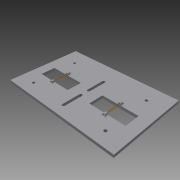
# Autodesk Inventor part: Down
Saved by Autodesk Inventor 2015 (Build 190159000, 159)
## iProperties
Created: 2018-12-21
Part Number: Down
Material: Типовые
Document SubType Name: Modeling
Designer: kostya
Density: 1 g/cm^3
Appearance: По умолчанию
Author: kostya
Autodesk Inventor part; units mm, degrees
ref_plane "YZ Plane" through (0, 0, 0) normal (1, 0, 0) x (0, 1, 0)
ref_plane "XZ Plane" through (0, 0, 0) normal (0, 1, 0) x (-1, 0, 0)
sketch "Эскиз1" plane through (0, 0, 0) normal (0, 0, 1) x (1, 0, 0)
  line L0 (-100, -75) -> (100, -75)
  line L1 (100, -75) -> (100, 75)
  line L2 (100, 75) -> (-100, 75)
  line L3 (-100, 75) -> (-100, -75)
  line L4 (-100, -75) -> (100, 75) construction
  line L5 (100, -75) -> (-100, 75) construction
  point P0 (0, 0)
  dimension "d0" = 200
  dimension "d1" = 150
  constraints: 12 end point, 2 midpoint, 2 parallel, 1 horizontal, 1 perpendicular
  measures "d0" distance of L2.end L1.end
  measures "d1" distance of L1.end L0.end
extrude "Выдавливание1" add sketch "Эскиз1" along normal blind 5
sketch "Эскиз2" plane through (0, 0, 5) normal (0, 0, 1) x (1, 0, 0)
  line L0 (-100, -75) -> (100, -75) projected
  line L1 (100, -75) -> (100, 75) projected
  line L2 (100, 75) -> (-100, 75) projected
  line L3 (-100, 75) -> (-100, -75) projected
  line L4 (100, 75) -> (-100, 75) construction
  line L5 (0, 75) -> (0, -75) construction
  line L6 (-100, 0) -> (100, 0) construction
  line L7 (100, -75) -> (100, 75) construction
  line L8 (-100, -12.5) -> (100, -12.5) construction
  line L9 (100, -12.5) -> (100, 12.5) construction
  line L10 (100, 12.5) -> (-100, 12.5) construction
  line L11 (-100, 12.5) -> (-100, -12.5) construction
  line L12 (-100, -12.5) -> (100, 12.5) construction
  line L13 (100, -12.5) -> (-100, 12.5) construction
  line L14 (-100, 0) -> (0, 0) construction
  line L15 (-51.2124, 75) -> (-51.2124, -75) construction
  line L16 (-100, -75) -> (100, -75) construction
  line L17 (0, 0) -> (100, 0) construction
  line L18 (50, 75) -> (50, -75) construction
  line L19 (-81.2124, -12.5) -> (-21.2124, -12.5)
  line L20 (-21.2124, -12.5) -> (-21.2124, 12.5)
  line L21 (-21.2124, 12.5) -> (-81.2124, 12.5)
  line L22 (-81.2124, 12.5) -> (-81.2124, -12.5)
  line L23 (-81.2124, -12.5) -> (-21.2124, 12.5) construction
  line L24 (-21.2124, -12.5) -> (-81.2124, 12.5) construction
  line L25 (81.2124, -12.5) -> (21.2124, -12.5)
  line L26 (21.2124, -12.5) -> (21.2124, 12.5)
  line L27 (21.2124, 12.5) -> (81.2124, 12.5)
  line L28 (81.2124, 12.5) -> (81.2124, -12.5)
  point P0 (-51.2124, 0)
  dimension "d4" = 25
  dimension "d5" = 60
  constraints: 44 end point, 9 midpoint, 6 point on line, 4 parallel, 4 perpendicular, 4 symmetric about line, 2 collinear, 2 horizontal
  measures "d4" distance of L9.end L8.end
  measures "d5" distance of L21.end L20.end
extrude "Выдавливание2" cut sketch "Эскиз2" against normal blind 5 contours L22 L21 L20 L19 | L25 L26 L27 L28
sketch "Эскиз3" plane through (-81.2124, 12.5, 5) normal (0, -1, 0) x (1, 0, 0)
  line L0 (0, 0) -> (60, 0) projected
  line L1 (30, 0) -> (30, 14.9537) construction
  line L2 (30, 0) -> (40, 0) construction
  line L3 (30, 0) -> (35, 0) construction
  line L4 (30, 0) -> (25, 0) construction
  line L5 (25, 0) -> (35, 0) construction
  line L6 (25, 0) -> (35, 0)
  line L7 (30, 0) -> (30, 3) construction
  circle A0 centre (30, 1.5) radius 1.5
  arc A1 (32.3946, 0.7816) -> (27.6054, 0.7816) centre (30, 1.5) ccw
  line L8 (35, 0) -> (32.3946, 0.7816)
  line L9 (25, 0) -> (27.6054, 0.7816)
  point P0 (81.2124, -5)
  dimension "d8" = 10
  dimension "d9" = 5
  dimension "d10" = 5
  dimension "d11" = 3
  dimension "d12" = 1
  constraints: 18 end point, 3 midpoint, 3 point on line, 2 collinear, 2 point on circle, 1 centre point, 1 vertical, 1 vertical alignment, 2 other
  measures "d8" distance of L1.start L2.end
  measures "d9" distance of L1.start L3.end
  measures "d10" distance of L1.start L4.end
  measures "d11" distance of L1.start L7.end
extrude "Выдавливание3" add sketch "Эскиз3" against normal blind 5
mirror "Зеркальное отражение1" about plane through (0, 0, 0) normal (0, 1, 0) of "Выдавливание3"
sketch "Эскиз4" plane through (-81.2124, 12.5, 0) normal (0, -1, 0) x (1, 0, 0)
  circle A0 centre (30, 6.5) radius 1.5 projected
  point P0 (81.2124, 0)
surface extrude "ВыдавПврх1" sketch "Эскиз4" along normal up to next shown yes curves A0
boundary_patch "Участок поверхности1"
boundary_patch "Участок поверхности2"
ref_plane "РабПлоскость1" through (-81.2124, 0, 0) normal (0, -1, 0) x (1, 0, 0)
sketch "Эскиз6" plane through (0, 0, 5) normal (0, 0, 1) x (1, 0, 0)
  line L0 (81.2124, -12.5) -> (21.2124, -12.5) projected
  line L1 (21.2124, -12.5) -> (21.2124, 12.5) projected
  line L2 (21.2124, 12.5) -> (81.2124, 12.5) projected
  line L3 (81.2124, 12.5) -> (81.2124, -12.5) projected
  line L4 (-100, -75) -> (100, -75) projected
  line L5 (100, -75) -> (100, 75) projected
  line L6 (100, 75) -> (-100, 75) projected
  line L7 (-100, 75) -> (-100, -75) projected
  line L8 (-46.2124, -12.5) -> (-46.2124, -17.5) projected
  line L9 (-46.2124, -17.5) -> (-51.2124, -17.5) projected
  line L10 (-51.2124, -17.5) -> (-56.2124, -17.5) projected
  line L11 (-56.2124, -17.5) -> (-56.2124, -12.5) projected
  line L12 (-56.2124, -12.5) -> (-81.2124, -12.5) projected
  line L13 (-81.2124, -12.5) -> (-81.2124, 12.5) projected
  line L14 (-81.2124, 12.5) -> (-56.2124, 12.5) projected
  line L15 (-56.2124, 12.5) -> (-56.2124, 17.5) projected
  line L16 (-56.2124, 17.5) -> (-51.2124, 17.5) projected
  line L17 (-51.2124, 17.5) -> (-46.2124, 17.5) projected
  line L18 (-46.2124, 17.5) -> (-46.2124, 12.5) projected
  line L19 (-46.2124, 12.5) -> (-21.2124, 12.5) projected
  line L20 (-21.2124, 12.5) -> (-21.2124, -12.5) projected
  line L21 (-21.2124, -12.5) -> (-46.2124, -12.5) projected
  line L22 (-100, -75) -> (100, -75) construction
  line L23 (-21.2124, -75) -> (-21.2124, 75) construction
  line L24 (100, 75) -> (-100, 75) construction
  line L25 (-21.2124, 12.5) -> (-21.2124, 75) construction
  line L26 (-21.2124, 75) -> (21.2124, 75) construction
  line L27 (21.2124, 75) -> (21.2124, 12.5) construction
  line L28 (21.2124, 12.5) -> (-21.2124, 12.5) construction
  line L29 (-21.2124, 12.5) -> (-21.2124, 75) construction
  line L30 (-21.2124, -75) -> (21.2124, -75) construction
  line L31 (21.2124, -75) -> (21.2124, -12.5) construction
  line L32 (21.2124, -12.5) -> (-21.2124, -12.5) construction
  line L33 (-21.2124, -12.5) -> (-21.2124, -75) construction
  line L34 (100, -75) -> (100, 75) construction
  line L35 (-100, -7.5) -> (100, -7.5) construction
  line L36 (100, -7.5) -> (100, 7.5) construction
  line L37 (100, 7.5) -> (-100, 7.5) construction
  line L38 (-100, 7.5) -> (-100, -7.5) construction
  line L39 (-100, -7.5) -> (100, 7.5) construction
  line L40 (100, -7.5) -> (-100, 7.5) construction
  line L41 (0, 7.5) -> (0, 17.5) construction
  line L42 (0, -7.5) -> (0, -28.0993) construction
  line L43 (-2.5, -7.5) -> (-2.5, -28.0993)
  line L44 (2.5, -28.0993) -> (2.5, -7.5)
  arc A0 (2.5, -7.5) -> (-2.5, -7.5) centre (0, -7.5) ccw
  line L45 (-2.5, -28.0993) -> (-2.5, -38.0993)
  line L46 (2.5, -28.0993) -> (2.5, -38.0993)
  arc A1 (-2.5, -38.0993) -> (2.5, -38.0993) centre (0, -38.0993) ccw
  line L47 (-21.2124, 0) -> (21.2124, 0) construction
  line L48 (-2.5, 7.5) -> (-2.5, 28.0993)
  line L49 (2.5, 28.0993) -> (2.5, 7.5)
  arc A2 (-2.5, 7.5) -> (2.5, 7.5) centre (0, 7.5) ccw
  line L50 (-2.5, 28.0993) -> (-2.5, 38.0993)
  line L51 (2.5, 28.0993) -> (2.5, 38.0993)
  arc A3 (2.5, 38.0993) -> (-2.5, 38.0993) centre (0, 38.0993) ccw
  point P0 (0, 0)
  point P1 (0, -17.7997)
  point P2 (0, 17.7997)
  dimension "d24" = 15
  dimension "d25" = 10
  dimension "d27" = 10
  constraints: 56 end point, 9 symmetric about line, 8 point on circle, 7 midpoint, 7 parallel, 4 centre point, 4 perpendicular, 4 vertical, 3 horizontal, 3 point on line, 1 coincident, 1 collinear, 2 other
  measures "d24" distance of L36.end L35.end
  measures "d25" distance of L41.start L41.end
  measures "d27" distance of L43.end L45.end
extrude "Выдавливание5" cut sketch "Эскиз6" against normal blind 20 contours A0 L44 L46 A1 L45 L43 | L48 L50 A3 L51 L49 A2
mirror "Зеркальное отражение2" about plane through (0, 0, 0) normal (1, 0, 0) of "Выдавливание3", "ВыдавПврх1", "Зеркальное отражение1"
sketch "Эскиз7" plane through (0, 0, 5) normal (0, 0, 1) x (1, 0, 0)
  arc A0 (-2.5, -38.0993) -> (2.5, -38.0993) centre (0, -38.0993) ccw projected
  line L0 (-2.5, -38.0993) -> (-2.5, -7.5) projected
  arc A1 (2.5, -7.5) -> (-2.5, -7.5) centre (0, -7.5) ccw projected
  line L1 (2.5, -7.5) -> (2.5, -38.0993) projected
  arc A2 (2.5, 38.0993) -> (-2.5, 38.0993) centre (0, 38.0993) ccw projected
  line L2 (2.5, 38.0993) -> (2.5, 7.5) projected
  arc A3 (-2.5, 7.5) -> (2.5, 7.5) centre (0, 7.5) ccw projected
  line L3 (-2.5, 7.5) -> (-2.5, 38.0993) projected
  line L4 (-100, -75) -> (100, -75) projected
  line L5 (100, -75) -> (100, 75) projected
  line L6 (100, 75) -> (-100, 75) projected
  line L7 (-100, 75) -> (-100, -75) projected
  line L8 (-46.2124, -12.5) -> (-46.2124, -17.5) projected
  line L9 (-46.2124, -17.5) -> (-51.2124, -17.5) projected
  line L10 (-51.2124, -17.5) -> (-56.2124, -17.5) projected
  line L11 (-56.2124, -17.5) -> (-56.2124, -12.5) projected
  line L12 (-56.2124, -12.5) -> (-81.2124, -12.5) projected
  line L13 (-81.2124, -12.5) -> (-81.2124, 12.5) projected
  line L14 (-81.2124, 12.5) -> (-56.2124, 12.5) projected
  line L15 (-56.2124, 12.5) -> (-56.2124, 17.5) projected
  line L16 (-56.2124, 17.5) -> (-51.2124, 17.5) projected
  line L17 (-51.2124, 17.5) -> (-46.2124, 17.5) projected
  line L18 (-46.2124, 17.5) -> (-46.2124, 12.5) projected
  line L19 (-46.2124, 12.5) -> (-21.2124, 12.5) projected
  line L20 (-21.2124, 12.5) -> (-21.2124, -12.5) projected
  line L21 (-21.2124, -12.5) -> (-46.2124, -12.5) projected
  line L22 (56.2124, -12.5) -> (56.2124, -17.5) projected
  line L23 (56.2124, -17.5) -> (51.2124, -17.5) projected
  line L24 (51.2124, -17.5) -> (46.2124, -17.5) projected
  line L25 (46.2124, -17.5) -> (46.2124, -12.5) projected
  line L26 (46.2124, -12.5) -> (21.2124, -12.5) projected
  line L27 (21.2124, -12.5) -> (21.2124, 12.5) projected
  line L28 (21.2124, 12.5) -> (46.2124, 12.5) projected
  line L29 (46.2124, 12.5) -> (46.2124, 17.5) projected
  line L30 (46.2124, 17.5) -> (51.2124, 17.5) projected
  line L31 (51.2124, 17.5) -> (56.2124, 17.5) projected
  line L32 (56.2124, 17.5) -> (56.2124, 12.5) projected
  line L33 (56.2124, 12.5) -> (81.2124, 12.5) projected
  line L34 (81.2124, 12.5) -> (81.2124, -12.5) projected
  line L35 (81.2124, -12.5) -> (56.2124, -12.5) projected
  line L36 (-100, 75) -> (-70, 75) construction
  line L37 (-70, 75) -> (-70, 45) construction
  line L38 (-70, 45) -> (-100, 45) construction
  line L39 (-100, 45) -> (-100, 75) construction
  circle A4 centre (-70, 45) radius 2.5
  line L40 (100, -75) -> (100, 75) construction
  line L41 (100, 0) -> (-100, 0) construction
  line L42 (100, 75) -> (-100, 75) construction
  line L43 (0, 75) -> (0, -75) construction
  line L44 (-100, -75) -> (100, -75) construction
  circle A5 centre (70, 45) radius 2.5
  line L45 (-100, -75) -> (100, -75) projected
  line L46 (-70, -75) -> (-70, -35) construction
  line L47 (-70, -35) -> (-100, -35) construction
  circle A6 centre (-70, -35) radius 2.5
  line L48 (70, -75) -> (70, -35) construction
  line L49 (70, -35) -> (100, -35) construction
  circle A7 centre (70, -35) radius 2.5
  line L50 (-100, -75) -> (-100, -55)
  line L51 (-100, -55) -> (100, -55)
  line L52 (100, -75) -> (100, -55)
  point P0 (0, 0)
  dimension "d30" = 30
  dimension "d31" = 30
  dimension "d32" = 5
  dimension "d35" = 40
  dimension "d36" = 5
  dimension "d37" = 20
  constraints: 26 end point, 6 symmetric about line, 5 perpendicular, 4 centre point, 4 coincident, 4 midpoint, 4 point on line, 2 parallel, 1 horizontal, 2 other
  measures "d30" distance of L37.end L38.end
  measures "d31" distance of L36.end L37.end
  measures "d32" diameter of A4
  measures "d35" distance of L46.start L46.end
  measures "d36" diameter of A6
  measures "d37" distance of L4.start L50.end
extrude "Выдавливание6" cut sketch "Эскиз7" against normal blind 20 contours L7 L51 L5 L4 | A4 | A5 | A6 | A7
body "SRF1"
body "SRF2"
body "SRF3"
body "SRF4"
